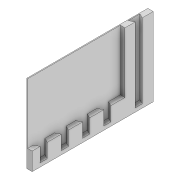
# Autodesk Inventor part: Sliding test receiver copy
Saved by Autodesk Inventor 2020 (Build 240168000, 168)
## iProperties
Created: 2019-11-10
Part Number: Sliding test receiver copy
Material: Generic
Document SubType Name: Modeling
Designer: ball
Density: 1 g/cm^3
Appearance: Default
Author: ball
Autodesk Inventor part; units mm, degrees
ref_plane "YZ Plane" through (0, 0, 0) normal (1, 0, 0) x (0, 1, 0)
ref_plane "XZ Plane" through (0, 0, 0) normal (0, 1, 0) x (-1, 0, 0)
ref_plane "XY Plane" through (0, 0, 0) normal (0, 0, 1) x (1, 0, 0)
sketch "Sketch1" plane through (0, 0, 0) normal (0, 1, 0) x (-1, 0, 0)
  line L0 (7.366, 0.1452) -> (7.366, -23.8548)
  line L1 (7.366, -23.8548) -> (0, -23.8548)
  line L2 (6.096, 4.754) -> (6.096, -4.754)
  line L3 (0, 4.754) -> (0, 7.802)
  line L4 (6.096, 7.802) -> (6.096, 4.754)
  line L5 (0, -4.754) -> (0, -7.548)
  line L6 (6.096, -7.802) -> (6.096, -4.754)
  line L7 (6.096, 7.802) -> (0, 4.754)
  line L8 (6.096, -7.802) -> (0, -4.754)
  line L9 (0, -23.8548) -> (0, -4.754)
  line L10 (0, 4.754) -> (0, 23.821)
  line L11 (6.096, 20.773) -> (6.096, 23.821)
  line L12 (6.096, 20.773) -> (0, 23.821)
  line L13 (6.096, 36.377) -> (6.096, 33.329)
  line L14 (6.096, 36.377) -> (0, 33.329)
  line L15 (6.096, 33.329) -> (6.096, 23.821)
  line L16 (6.096, 49.348) -> (6.096, 52.396)
  line L17 (6.096, 49.348) -> (0, 52.396)
  line L18 (6.096, 64.952) -> (6.096, 61.904)
  line L19 (6.096, 64.952) -> (0, 61.904)
  line L20 (6.096, 61.904) -> (6.096, 52.396)
  line L21 (6.096, 77.923) -> (6.096, 80.971)
  line L22 (6.096, 77.923) -> (0, 80.971)
  line L23 (6.096, 93.527) -> (6.096, 90.479)
  line L24 (6.096, 93.527) -> (0, 90.479)
  line L25 (6.096, 90.479) -> (6.096, 80.971)
  line L26 (7.366, 0.1452) -> (7.366, 101.147)
  line L27 (7.366, 101.147) -> (0, 101.147)
  line L28 (0, 33.329) -> (0, 52.396)
  line L29 (0, 61.904) -> (0, 80.971)
  line L30 (0, 90.479) -> (0, 101.147)
  point P0 (0, 0)
  dimension "d0" = 7.366
  dimension "d1" = 24
  dimension "d8" = 9.508
  dimension "d9" = 4.754
  dimension "d10" = 3.048
  dimension "d11" = 3.048
  dimension "d12" = 6.096
  dimension "d17" = 28.575
  dimension "d23" = 7.62
  dimension "d24" = 16.0528
  dimension "d31" = 125.0018
  constraints: 62 end point, 5 vertical, 4 parallel, 2 point on line, 1 horizontal, 33 other
  measures "d0" distance of L0.end L1.end
  measures "d1" distance of L0.start L0.end
  measures "d8" distance of L5.start L3.start
  measures "d9" distance of point (0, 0) L3.start
  measures "d10" vertical distance of L4.start L3.start
  measures "d11" vertical distance of L6.start L5.start
  measures "d12" distance from line of L9 L6.start
  measures "d17" distance of L2.end L11.end
  measures "d23" distance from line of L27 L23.start
  measures "d24" distance from line of L1 L6.start
  measures "d31" distance between parallel lines of L1 L27
extrude "MultipleTeeth" add sketch "Sketch1" along normal blind 19.05
sketch "Sketch2" plane through (0, 0, 0) normal (0, -1, 0) x (1, 0, 0)
  line L0 (0, 4.754) -> (-6.096, 7.802) construction
  line L1 (-6.096, 7.802) -> (-6.096, -7.802) construction
  line L2 (-6.096, -7.802) -> (0, -4.754) construction
  line L3 (0, 23.821) -> (0, 4.754) projected
  line L4 (0, 4.754) -> (-6.096, 7.802)
  line L5 (-6.096, -7.802) -> (0, -4.754) projected
  line L6 (-6.096, 7.802) -> (-6.096, -7.802) projected
  line L7 (-6.096, -7.802) -> (-6.096, 7.802)
  line L8 (0, -4.754) -> (-6.096, -7.802)
  line L9 (-7.366, -23.8548) -> (-7.366, 101.147) projected
  line L10 (-7.366, -59.508) -> (-7.366, -32.8548)
  line L11 (-7.366, -23.8548) -> (0, -23.8548)
  line L12 (-7.366, 101.147) -> (0, 101.147) projected
  line L13 (-7.366, -55.8503) -> (-7.366, -40.458) construction
  line L14 (0, -43.0234) -> (0, -59.508) construction
  line L15 (-6.096, -62.0648) -> (0, -62.0648) construction
  line L16 (0, -32.8548) -> (0, -37.6258)
  line L17 (0, -49.9828) -> (0, -62.0648)
  line L18 (0, -62.0648) -> (0, -59.508)
  line L19 (0, -32.8548) -> (-7.366, -32.8548) construction
  line L20 (0, -51.9048) -> (-7.366, -51.9048) construction
  line L21 (0, -42.3798) -> (-7.366, -42.3798) construction
  line L22 (-6.096, -7.802) -> (-6.096, -62.0648) construction
  line L23 (0, -37.6258) -> (-6.096, -34.5778)
  line L24 (-6.096, -50.1818) -> (-6.096, -34.5778)
  line L25 (0, -47.1338) -> (-6.096, -50.1818)
  line L26 (0, -4.754) -> (0, -23.8548) projected
  line L27 (0, -23.8548) -> (0, -32.8548)
  line L28 (-7.366, -32.8548) -> (-7.366, -23.8548)
  line L29 (0, -49.9828) -> (0, -47.1338)
  line L30 (0, -62.0648) -> (-7.366, -62.0648)
  line L31 (-7.366, -62.0648) -> (-7.366, -59.508)
  point P0 (0, 0)
  dimension "d25" = 125.0018
  dimension "d33" = 9
  dimension "d34" = 19.05
  dimension "d36" = 9.525
  dimension "d38" = 10.16
  constraints: 46 end point, 4 parallel, 4 perpendicular, 4 point on line, 3 collinear, 2 horizontal, 2 vertical
  measures "d25" distance between parallel lines of L12 L11
  measures "d33" distance of L16.start L11.end
  measures "d34" distance between parallel lines of L20 L19
  measures "d36" distance between parallel lines of L21 L19
  measures "d38" distance between parallel lines of L15 L20
extrude "LongTooth" add sketch "Sketch2" against normal blind 100.2792
sketch "Sketch3" plane through (0, 19.05, 0) normal (0, 1, 0) x (1, 0, 0)
  line L0 (-6.096, -7.802) -> (-6.096, 7.802) construction
  line L1 (0, 23.8548) -> (-7.366, 23.8548) projected
  line L2 (-7.366, -101.147) -> (0, -101.147) projected
  line L3 (-7.366, 23.8548) -> (-6.096, 23.8548)
  line L4 (-6.096, 23.8548) -> (-6.096, -101.147)
  line L5 (-6.096, -101.147) -> (-7.366, -101.147)
  line L6 (-7.366, -101.147) -> (-7.366, 23.8548)
  point P0 (0, 0)
  constraints: 8 end point, 2 parallel, 1 horizontal, 1 perpendicular, 1 point on line
extrude "ThinPlate" add sketch "Sketch3" along normal up to surface (81.2292 mm away)
sketch "Sketch4" plane through (0, 0, 0) normal (0, -1, 0) x (1, 0, 0)
  line L0 (-6.096, 101.147) -> (0, 101.147) projected
  line L1 (-7.366, 101.147) -> (-7.366, -62.0648) projected
  line L2 (0, 101.147) -> (-7.366, 101.147)
  line L3 (-7.366, 101.147) -> (-7.366, -62.0648)
  line L4 (-7.366, -62.0648) -> (0, -62.0648)
  line L5 (0, -62.0648) -> (0, 101.147)
  point P0 (0, 0)
  constraints: 8 end point, 2 parallel, 1 horizontal, 1 perpendicular
extrude "Extrusion4" add sketch "Sketch4" along normal blind 5.08
equation "\"d9\" = 0.5 * d8"
equation "\"d11\" = d10"
equation "\"d36\" = 0.5 * d34"
body "Solid1"
